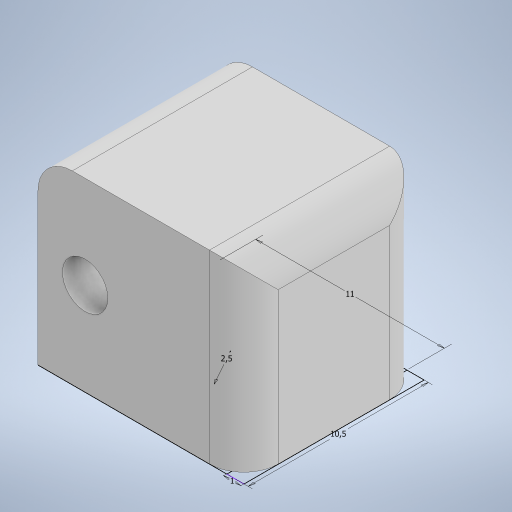
# Autodesk Inventor part: pusher
Saved by Autodesk Inventor 2023 (Build 270158000, 158)
## iProperties
Created: 2026-02-18
Part Number: pusher
Material: Типовые
Document SubType Name: Modeling
Designer: garin
Density: 1 g/cm^3
Appearance: По умолчанию
Author: garin
Autodesk Inventor part; units mm, degrees
ref_plane "YZ Plane" through (0, 0, 0) normal (1, 0, 0) x (0, 1, 0)
ref_plane "XZ Plane" through (0, 0, 0) normal (0, 1, 0) x (-1, 0, 0)
ref_plane "XY Plane" through (0, 0, 0) normal (0, 0, 1) x (1, 0, 0)
sketch "Эскиз2" plane through (0, 0, 0) normal (0, 1, 0) x (-1, 0, 0)
  line L0 (5.5, 5.25) -> (-5.5, 5.25)
  line L1 (-5.5, 5.25) -> (-5.5, -5.25)
  line L2 (-5.5, -5.25) -> (5.5, -5.25)
  line L3 (5.5, -5.25) -> (5.5, 5.25)
  line L4 (5.5, 0) -> (-5.5, 0) construction
  line L5 (0, 5.25) -> (0, -5.25) construction
  circle A0 centre (0, 0) radius 1.25
  line L6 (-5.5, -5.25) -> (-6.5, -5.25)
  line L7 (-6.5, -5.25) -> (-6.5, 5.25)
  line L8 (-6.5, 5.25) -> (-5.5, 5.25)
  line L9 (-5.5, 5.25) -> (-5.5, -5.25)
  dimension "d0" = 11
  dimension "d1" = 10.5
  dimension "d2" = 2.5
  dimension "d12" = 1
  constraints: 20 end point, 5 midpoint, 4 parallel, 2 coincident, 2 horizontal, 2 perpendicular, 1 centre point
  measures "d0" distance of L2.end L1.end
  measures "d1" distance of L1.end L0.end
  measures "d2" diameter of A0
  measures "d12" distance of L7.end L8.end
extrude "Выдавливание1" add sketch "Эскиз2" along normal blind 10.8 contours L3 L2 L1 L0 | L1 L6 L7 L8 | A0
sketch "Эскиз4" plane through (-5.5, 0, 5.25) normal (0, 0, 1) x (1, 0, 0)
  line L0 (5.5, 0) -> (2.75, 10.8) construction
  line L1 (5.5, 10.8) -> (0, 10.8) construction
  line L2 (0, 0) -> (0, 10.8) construction
  line L3 (0, 5.4) -> (5.5, 5.4) construction
  line L4 (5.5, 0) -> (5.5, 10.8) construction
  circle A0 centre (2.75, 5.4) radius 1.325
  dimension "d8" = 2.65
  constraints: 4 end point, 4 midpoint, 1 centre point
  measures "d8" diameter of A0
extrude "Выдавливание3" cut sketch "Эскиз4" against normal blind 10.5
fillet "Сопряжение2" radius 2 4 edges at (6.5, 5.4, 5.25) (6.5, 5.4, -5.25) (6.5, 10.8, 0) (-5.5, 10.8, 0)
